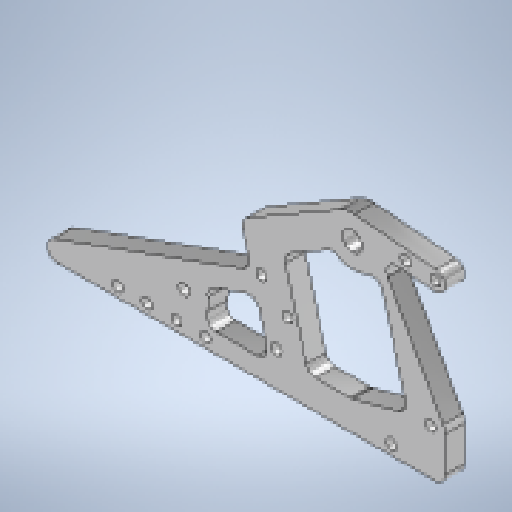
# Autodesk Inventor part: Uprights
Saved by Autodesk Inventor 2023.2 (Build 272271000, 271)
## iProperties
Created: 2024-01-11
Part Number: Uprights
Material: Aluminum 6061
Document SubType Name: Modeling
Designer: Nathan Cai
Mass: 48.3037 g
Surface Area: 101.197 cm^2
Volume: 17.8903 cm^3
Density: 2.7 g/cm^3
Appearance: Aluminum - Flat
Angle_Mount: 105.00 deg
Rail_Offset: 1.438 in
Author: Nathan Cai
Autodesk Inventor part; units mm, degrees
ref_plane "YZ Plane" through (0, 0, 0) normal (1, 0, 0) x (0, 1, 0)
ref_plane "XZ Plane" through (0, 0, 0) normal (0, 1, 0) x (-1, 0, 0)
ref_plane "XY Plane" through (0, 0, 0) normal (0, 0, 1) x (1, 0, 0)
sketch "Sketch2" plane through (0, 0, 0) normal (0, 0, 1) x (1, 0, 0)
  circle A0 centre (0, 0) radius 3.175
  circle A1 centre (0, 0) radius 7.9375
  line L0 (-24.9815, -53.975) -> (30.0677, -53.975)
  line L1 (-24.9815, -53.975) -> (-36.2864, -11.7845)
  line L2 (-36.2864, -11.7845) -> (-3.9688, 6.8741)
  line L3 (20.5427, -47.625) -> (-13.5349, -47.625)
  line L4 (-13.5349, -47.625) -> (-22.3476, -14.7355)
  line L5 (-22.3476, -14.7355) -> (-5.9414, -5.2634)
  line L6 (-18.5621, -41.1307) -> (-23.4926, -22.7298) construction
  line L7 (-23.4926, -22.7298) -> (-29.6262, -24.3733) construction
  line L8 (-29.6262, -24.3733) -> (-24.6957, -42.7742) construction
  line L9 (-24.6957, -42.7742) -> (-18.5621, -41.1307) construction
  line L10 (-18.5621, -41.1307) -> (-29.6262, -24.3733) construction
  line L11 (-23.4926, -22.7298) -> (-24.6957, -42.7742) construction
  circle A2 centre (-29.6262, -24.3733) radius 1.7526
  circle A3 centre (-24.6957, -42.7742) radius 1.7526
  circle A4 centre (-21.0273, -31.9303) radius 1.7526
  line L12 (25.3052, -45.5804) -> (25.3052, -53.975) construction
  circle A5 centre (25.3052, -39.2375) radius 1.7526
  line L13 (0, 0) -> (-58.6646, -15.7191) construction
  line L14 (-24.0941, -32.752) -> (-30.6681, -8.2175) construction
  circle A6 centre (25.3052, -39.2375) radius 4.7625
  line L15 (30.0677, -39.2375) -> (30.0677, -53.975)
  line L16 (20.5427, -39.2375) -> (20.5427, -47.625)
  line L17 (-30.2278, -34.3955) -> (-17.9605, -31.1085) construction
  line L18 (-24.9815, -53.975) -> (-113.8815, -53.975)
  circle A7 centre (-9.9632, -48.6877) radius 1.7526
  line L19 (-9.9632, -48.6877) -> (-25.2973, -52.7964) construction
  line L20 (25.3052, -39.2375) -> (24.0725, -34.6373) construction
  line L21 (-31.2313, -30.6503) -> (-77.8688, -47.625)
  line L22 (-77.8688, -47.625) -> (-26.6829, -47.625)
  line L23 (-9.9632, -48.6877) -> (-10.4168, -46.9948) construction
  circle A8 centre (25.3052, -39.2375) radius 1.7526
  circle A9 centre (25.3052, -39.2375) radius 4.7625
  line L24 (17.994, -39.5531) -> (8.9547, -5.8181)
  line L25 (8.9547, -5.8181) -> (-22.4801, -14.241) construction
  line L26 (-22.4801, -14.241) -> (-13.4409, -47.976) construction
  line L27 (-0.2817, -44.45) -> (17.994, -39.5531)
  line L28 (17.994, -39.5531) -> (-22.4801, -14.241) construction
  line L29 (8.9547, -5.8181) -> (-13.4409, -47.976) construction
  line L30 (6.9477, 3.8384) -> (29.4738, -36.9345)
  line L31 (2.0544, -7.667) -> (8.9547, -5.8181)
  circle A10 centre (-9.9632, -48.6877) radius 4.7625 construction
  line L32 (-0.2817, -44.45) -> (-14.3857, -44.45)
  line L33 (-113.8815, -53.975) -> (-32.8811, -24.4933)
  circle A11 centre (-54.7623, -40.9695) radius 1.7526
  circle A12 centre (-54.7623, -40.9695) radius 7.9375
  line L34 (-54.7623, -40.9695) -> (-56.8404, -33.2138) construction
  line L35 (-25.8322, -50.8) -> (-105.1582, -50.8) construction
  circle A13 centre (-47.625, -50.8) radius 1.7526
  circle A14 centre (-57.15, -50.8) radius 1.7526
  circle A15 centre (-66.675, -50.8) radius 1.7526
  circle A16 centre (-76.2, -50.8) radius 1.7526
  circle A17 centre (12.7, -50.8) radius 1.7526
  line L36 (0.6918, 7.9073) -> (27.1694, 5.5908)
  circle A18 centre (26.8927, 2.4279) radius 1.7526
  circle A19 centre (26.8927, 2.4279) radius 3.175
  line L37 (8.6038, 0.8408) -> (26.616, -0.735)
  circle A20 centre (17.4039, 3.258) radius 1.7526
  line L38 (-9.9632, -48.6877) -> (-9.9632, -48.6877) construction
  point P0 (7.667, 2.0544)
  point P1 (0.4795, -7.923)
  point P2 (-24.0941, -32.752)
  point P3 (-2.2431, -26.897)
  point P4 (-2.2431, -26.897)
  point P5 (-12.1309, -47.625)
  point P6 (-15.5208, -47.3441)
  point P7 (29.4738, -36.9345)
  point P8 (-14.3857, -44.45)
  point P9 (-9.6568, -46.9621)
  point P10 (-9.6568, -46.9621)
  point P11 (-48.0301, -36.7646)
  point P12 (-59.0876, -47.625)
  point P13 (-62.6223, -42.0757)
  point P14 (-50.4369, -47.625)
  point P15 (13.8439, -8.6439)
  point P16 (24.4605, 0.387)
  point P17 (23.7298, 2.7046)
  dimension "d7" = 15.875
  dimension "d40" = 3.5052
  dimension "d6" = 6.35
  dimension "Angle_Mount" = 105
  dimension "d17" = 105
  dimension "d19" = 9.525
  dimension "d20" = 12.7
  dimension "d24" = 19.05
  dimension "d25" = 6.35
  dimension "d26" = 3.5052
  dimension "d27" = 3.5052
  dimension "d28" = 3.5052
  dimension "d29" = 6.35
  dimension "d33" = 3.5052
  dimension "d35" = 31.75
  dimension "d37" = 9.525
  dimension "d38" = 25.4
  dimension "d39" = 53.975
  dimension "d41" = 44.45
  dimension "Rail_Offset" = 36.5125
  dimension "d45" = 6.35
  dimension "d48" = 22.225
  dimension "d49" = 3.5052
  dimension "d51" = 9.525
  dimension "d52" = 32.5438
  dimension "d53" = 34.925
  dimension "d54" = 9.525
  dimension "d56" = 9.525
  dimension "d58" = 6.35
  dimension "d60" = 20
  dimension "d61" = 88.9
  dimension "d69" = 31.75
  dimension "d71" = 3.5052
  dimension "d72" = 15.875
  dimension "d74" = 3.175
  dimension "d75" = 3.5052
  dimension "d76" = 47.625
  dimension "d79" = 9.525
  dimension "d84" = 3.5052
  dimension "d85" = 60.325
  dimension "d86" = 145
  dimension "d87" = 3.5052
  dimension "d88" = 6.35
  dimension "d101" = 9.525
  constraints: 78 end point, 23 point on line, 19 centre point, 12 parallel, 11 perpendicular, 10 coincident, 10 point on circle, 8 midpoint, 6 tangent, 3 horizontal, 1 collinear, 1 concentric, 25 other
  measures "d6" diameter of A0
  measures "Angle_Mount" angle of L0 L1
  measures "d17" angle of L2 L1
  measures "d19" distance between parallel lines of L2 L5
  measures "d20" distance between parallel lines of L1 L4
  measures "d24" distance of L6.start L6.end
  measures "d25" distance of L7.end L6.end
  measures "d26" diameter of A2
  measures "d27" diameter of A3
  measures "d28" diameter of A4
  measures "d29" distance between parallel lines of L0 L3
  measures "d33" diameter of A5
  measures "d35" distance from line of point (0, 0) L14
  measures "d37" diameter of A6
  measures "d38" distance between parallel lines of L13 L17
  measures "d39" distance from line of L0 point (0, 0)
  measures "d41" distance between parallel lines of L13 L19
  measures "Rail_Offset" distance from line of L19.start L20
  measures "d45" distance between parallel lines of L18 L22
  measures "d48" distance from line of point (0, 0) L23
  measures "d49" diameter of A8
  measures "d51" diameter of A9
  measures "d52" distance between parallel lines of L24 L26
  measures "d53" distance between parallel lines of L27 L25
  measures "d54" diameter of A10
  measures "d56" distance between parallel lines of L0 L32
  measures "d58" distance between parallel lines of L21 L33
  measures "d60" angle of L22 L21
  measures "d61" distance of L0.start L18.end
  measures "d69" distance between parallel lines of L14 L34
  measures "d71" diameter of A11
  measures "d72" diameter of A12
  measures "d74" distance between parallel lines of L22 L35
  measures "d75" diameter of A13
  measures "d76" horizontal distance of A13.centre L13.start
  measures "d79" distance of A13.centre A14.centre
  measures "d84" diameter of A17
  measures "d85" distance of A13.centre A17.centre
  measures "d86" angle of L2 L36
  measures "d87" diameter of A18
  measures "d88" diameter of A19
  measures "d101" distance of A18.centre A20.centre
extrude "Extrusion2" add sketch "Sketch2" along normal blind 6.35 contours A1 | A1 L30 A6 L16 L3 A7 L4 L32 L27 L24 L31 | A1 L36 A19 L37 L30 | L5 L4 L3 A7 L16 A6 L15 L0 L1 L2 A1 | A19 | A6 | L1 L21 A12 L22 L18 L33 | A7 L3 | L3 A7 | A12 L22 L21 A11 | L21 A11 A12 | A12 L22 | A12 L22 L21
fillet "Fillet1" radius 3.175 15 edges at (-22.3476, -14.7355, 3.175) (-5.9414, -5.2634, 3.175) (8.9547, -5.8181, 3.175) (17.994, -39.5531, 3.175) (-14.3857, -44.45, 3.175) (-0.2817, -44.45, 3.175) (30.0677, -53.975, 3.175) (-36.2864, -11.7845, 3.175) (-26.6829, -47.625, 3.175) (-50.4369, -47.625, 3.175) (-48.0301, -36.7646, 3.175) (-31.2313, -30.6503, 3.175) (-32.8811, -24.4933, 3.175) (-113.8815, -53.975, 3.175) (8.6038, 0.8408, 3.175)
body "Solid2"
